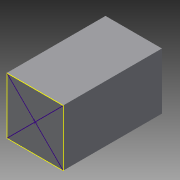
# Autodesk Inventor part: 知能ロボコンボールキャスタ
Saved by Autodesk Inventor 2013 (Build 170138000, 138)
## iProperties
Created: 2014-05-11
Part Number: 知能ロボコンボールキャスタ
Material: 一般
Document SubType Name: Modeling
Designer: horumo136
Density: 1 g/cm^3
Author: horumo136
Autodesk Inventor part; units mm, degrees
ref_plane "YZ Plane" through (0, 0, 0) normal (1, 0, 0) x (0, 1, 0)
ref_plane "XZ Plane" through (0, 0, 0) normal (0, 1, 0) x (-1, 0, 0)
ref_plane "XY Plane" through (0, 0, 0) normal (0, 0, 1) x (1, 0, 0)
sketch "スケッチ1" plane through (0, 0, 0) normal (0, 1, 0) x (-1, 0, 0)
  line L0 (0, 0) -> (-20, 0)
  line L1 (-20, 0) -> (-20, 20)
  line L2 (-20, 20) -> (0, 20)
  line L3 (0, 20) -> (0, 0)
  dimension "d0" = 20
  dimension "d1" = 20
  constraints: 8 end point, 2 parallel, 1 horizontal, 1 perpendicular
  measures "d0" distance of L1.end L2.end
  measures "d1" distance of L0.end L1.end
extrude "押し出し1" add sketch "スケッチ1" along normal blind 35
sketch "スケッチ2" plane through (0, 35, 0) normal (0, 1, 0) x (1, 0, 0)
  line L0 (20, 0) -> (0, 0) projected
  line L1 (0, 0) -> (0, -20) projected
  line L2 (0, -20) -> (20, -20) projected
  line L3 (20, -20) -> (20, 0) projected
  line L4 (0, -10) -> (20, -10)
  line L5 (10, 0) -> (10, -20)
  circle A0 centre (10, -10) radius 4
  line L6 (12.4988, -13.1235) -> (7.5012, -6.8765)
  dimension "d4" = 8
  constraints: 6 end point, 6 midpoint, 2 point on circle, 1 centre point, 1 coincident
  measures "d4" diameter of A0
revolve "回転1" add sketch "スケッチ2" angle 360 about axis through (12.4988, 35, 13.1235) along (-0.6246951, 0, -0.7808688) picked at (12.2437, -8.5902) picked at (8.5873, -7.7581) picked at (11.8763, -11.8713) contours A0 L4 L5 | L5 L6 A0 | A0 L6 L4
sketch "スケッチ3" plane through (0, 0, 0) normal (0, -1, 0) x (1, 0, 0)
  line L0 (0, 0) -> (20, 0) projected
  line L1 (20, 0) -> (20, 20) projected
  line L2 (20, 20) -> (0, 20) projected
  line L3 (0, 20) -> (0, 0) projected
  line L4 (20, 20) -> (0, 0)
  line L5 (0, 20) -> (20, 0)
  point P0 (10, 10)
  constraints: 4 end point, 1 midpoint, 1 perpendicular
